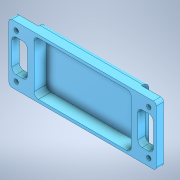
# Autodesk Inventor part: BodyStructure Front
Saved by Autodesk Inventor 2022.2 (Build 262287000, 287)
## iProperties
Created: 2019-11-06
Part Number: BodyStructure Front
Material: solidworks materials|ABS
Document SubType Name: Modeling
Designer: Jochen
Density: 1.02 g/cm^3
Appearance: 255,255,255
Sending System: SolidWorks 2017
Last Author: Felix
Last Saved: 2021-02-23
Author: Jochen
Autodesk Inventor part; units mm, degrees
ref_plane "YZ Plane" through (0, 0, 0) normal (1, 0, 0) x (0, 1, 0)
ref_plane "XZ Plane" through (0, 0, 0) normal (0, 1, 0) x (-1, 0, 0)
ref_plane "XY Plane" through (0, 0, 0) normal (0, 0, 1) x (1, 0, 0)
sketch "Sketch1" plane through (0, 0, 0) normal (0, 0, 1) x (1, 0, 0)
  line L0 (0, -28) -> (0, 28) construction
  line L1 (-70, 0) -> (70, 0) construction
  line L2 (-50, -20) -> (50, -20)
  line L3 (50, -20) -> (50, 20)
  line L4 (50, 20) -> (-50, 20)
  line L5 (-50, 20) -> (-50, -20)
  line L6 (-48, -11) -> (-37.5, -11)
  line L7 (-37.5, -11) -> (-37.5, 11)
  line L8 (-37.5, 11) -> (-48, 11)
  line L9 (-48, 11) -> (-48, -11)
  line L10 (37.5, -11) -> (48, -11)
  line L11 (48, -11) -> (48, 11)
  line L12 (48, 11) -> (37.5, 11)
  line L13 (37.5, 11) -> (37.5, -11)
  line L14 (-33, -18) -> (-33, 18)
  line L15 (33, 18) -> (33, -18)
  circle A0 centre (-45, -15) radius 1.5
  circle A1 centre (-45, 15) radius 1.5
  circle A2 centre (45, 15) radius 1.5
  circle A3 centre (45, -15) radius 1.5
  line L16 (-45, -15) -> (45, -15) construction
  line L17 (45, -15) -> (45, 15) construction
  line L18 (45, 15) -> (-45, 15) construction
  line L19 (-45, 15) -> (-45, -15) construction
  line L20 (-50, 0) -> (50, 0) construction
  line L21 (-33, 18) -> (33, 18)
  line L22 (-33, -18) -> (33, -18)
  line L23 (-35, 20) -> (-35, -20)
  line L24 (35, 20) -> (35, -20)
  point P0 (0, 0)
  point P1 (33, -11)
  dimension "d0" = 22
  dimension "d1" = 3
  dimension "d2" = 10.5
  dimension "d3" = 40
  dimension "d4" = 100
  dimension "d5" = 2
  dimension "d6" = 66
  dimension "d7" = 90
  dimension "d8" = 30
  dimension "d14" = 36
  dimension "d15" = 70
  constraints: 46 end point, 10 parallel, 6 horizontal, 6 perpendicular, 5 point on line, 4 centre point, 3 equal radius, 3 midpoint, 2 coincident, 2 equal length, 1 collinear, 8 other
  measures "d0" distance of L10.end L11.end
  measures "d1" diameter of A3
  measures "d2" distance between parallel lines of L11 L13
  measures "d3" distance of L2.end L3.end
  measures "d4" distance of L3.end L4.end
  measures "d5" distance from line of L20.end L11
  measures "d6" distance between parallel lines of L15 L14
  measures "d7" distance of L17.end L18.end
  measures "d8" distance of L18.end L16.start
  measures "d14" distance of L14.start L14.end
  measures "d15" distance between parallel lines of L24 L23
extrude "Extrusion1" add sketch "Sketch1" against normal blind 10 contours L5 L4 L23 L2 | L23 L4 L24 L2 | L24 L4 L3 L2 | L14 L21 L15 L22
extrude "Extrusion2" cut sketch "Sketch1" against normal blind 8.5 contours L14 L21 L15 L22
extrude "Extrusion3" cut sketch "Sketch1" along normal blind 5 from surface at -10 contours L5 L4 L23 L2 | L24 L4 L3 L2
fillet "Fillet1" radius 2 4 edges at (50, 20, -2.5) (50, -20, -2.5) (-50, 20, -2.5) (-50, -20, -2.5)
fillet "Fillet2" radius 3 12 edges at (-37.5, -11, -2.5) (-48, -11, -2.5) (37.5, -11, -2.5) (48, -11, -2.5) (48, 11, -2.5) (37.5, 11, -2.5) (-48, 11, -2.5) (-37.5, 11, -2.5) (-33, 18, -4.25) (33, 18, -4.25) (-33, -18, -4.25) (33, -18, -4.25)
fillet "Fillet3" radius 4 2 edges at (0, 20, -10) (0, -20, -10)
body "Solid1"
body "Solid2"
